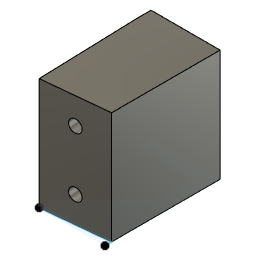
Wanhao-dub-D6-switchholder v3 (Autodesk Fusion 360 design; units mm, degrees)
Autodesk Fusion 360 part; units mm, degrees
note: some values were not read from the file. Set by a fixed rule: which sketch regions a step uses.
sketch "Sketch1" plane through (0, 0, 0) normal (0, 1, 0) x (1, 0, 0)
  line L0 (10, -10) -> (26, -10)
  line L1 (26, -10) -> (26, -50)
  line L2 (26, -50) -> (10, -50)
  line L3 (10, -50) -> (10, -10)
  line L4 (50, -25) -> (70, -25)
  line L5 (70, -25) -> (70, -55)
  line L6 (70, -55) -> (50, -55)
  line L7 (50, -55) -> (50, -25)
  line L8 (70, -25) -> (66, -25)
  line L9 (66, -25) -> (66, -55)
  line L10 (66, -55) -> (70, -55)
  line L11 (70, -55) -> (70, -25)
  dimension "d1" = 16
  dimension "d2" = 40
  dimension "d3" = 20
  dimension "d4" = 30
  dimension "d5" = 4
  dimension "d6" = 16
  constraint horizontal L0
  constraint vertical L1
  constraint horizontal L2
  constraint vertical L3
  constraint horizontal L4
  constraint vertical L5
  constraint horizontal L6
  constraint vertical L7
  constraint horizontal L8
  constraint vertical L9
  constraint horizontal L10
  constraint vertical L11
  measures "d1" distance of L0.start L0.end
  measures "d2" distance of L0.start L2.end
  measures "d3" distance of L4.start L4.end
  measures "d4" distance of L4.start L6.end
  measures "d5" distance of L4.end L8.end
  measures "d6" distance of L7 L9
extrude "Extrude1" add sketch "Sketch1" along normal blind 4 contours L4 L6 L7 L9 makes body 1
extrude "Extrude2" add sketch "Sketch1" along normal blind 35 contours L4 L5 L6 L8 L9 L10 L11 bodies 1
move_body "Move1" bodies 1 to x (1, 0, 0) y (0, 1, 0) z (0, 0, 1) at (-50, 0, -25)
sketch "Sketch2" plane through (16, 0, 0) normal (-1, 0, 0) x (0, 0, 1)
  line L0 (0, 4) -> (30, 4)
  line L1 (30, 4) -> (30, 35)
  line L2 (30, 35) -> (0, 35)
  line L3 (0, 35) -> (0, 4)
  line L4 (0, 35) -> (30, 35)
  line L5 (30, 35) -> (30, 31)
  line L6 (30, 31) -> (0, 31)
  line L7 (0, 31) -> (0, 35)
  dimension "d14" = 4
  constraint horizontal L4
  constraint vertical L5
  constraint horizontal L6
  constraint vertical L7
  constraint coincident L2.end L3.start
  measures "d14" distance of L2.end L6.end
extrude "Extrude3" add sketch "Sketch2" along normal blind 16 contours L1 L2 L3 L4 L5 L6 L7 bodies 1
move_body "Move2" bodies 1 to x (1, 0, 0) y (0, 0, 1) z (0, -1, 0) at (0, 30, 0)
sketch "Sketch3" plane through (0, 30, 0) normal (0, 1, 0) x (-1, 0, 0)
  line L0 (-20, 0) -> (0, 0)
  line L1 (0, 0) -> (0, 4)
  line L2 (0, 4) -> (-16, 4)
  line L3 (-16, 4) -> (-16, 31)
  line L4 (-16, 31) -> (0, 31)
  line L5 (0, 31) -> (0, 35)
  line L6 (0, 35) -> (-20, 35)
  line L7 (-20, 35) -> (-20, 0)
  line L8 (-16, 31) -> (0, 31)
  line L9 (-16, 15) -> (-16, 31)
  line L10 (-16, 15) -> (0, 31)
  dimension "d17" = 16
  constraint horizontal L8
  constraint vertical L9
  constraint coincident L3.end L4.start
  constraint coincident L4.end L5.start
  measures "d17" distance of L3.end L9.start
extrude "Extrude4" add sketch "Sketch3" against normal blind 30 separate body contours L3 L4 L8 L9 L10 makes body 2
move_face "OffsetFaces1" offset 1 1 faces at (0, 10, 1.3333) on bodies 1
sketch "Sketch4" plane through (0, 0, 4) normal (0, 0, 1) x (1, 0, 0)
  line L0 (16, 30) -> (-1, 30)
  line L1 (-1, 30) -> (-1, 0)
  line L2 (-1, 0) -> (16, 0)
  line L3 (16, 0) -> (16, 30)
  line L4 (-1, 30) -> (2, 30)
  line L5 (2, 30) -> (2, 0)
  line L6 (2, 30) -> (2, 26)
  line L7 (2, 26) -> (2, 7)
  circle A0 centre (2, 26) radius 1.5
  circle A1 centre (2, 7) radius 1.5
  dimension "d21" = 3
  dimension "d22" = 4
  dimension "d23" = 19
  dimension "d24" = 3
  dimension "d25" = 3
  constraint coincident L0.end L1.start
  constraint perpendicular L1 L4
  constraint coincident L2 L5.end
  constraint perpendicular L2 L5
  constraint perpendicular L4 L6
  constraint parallel L5 L7
  constraint coincident L6.end L7.start
  constraint coincident L7.end A1.centre
  measures "d21" distance of L0.end L4.end
  measures "d22" distance of L4.end L6.end
  measures "d23" distance of L6.end L7.end
  measures "d24" diameter of A0
  measures "d25" diameter of A1
extrude "Extrude5" cut sketch "Sketch4" against normal blind 6.6 contours L5 L6 L7 A0 | L5 L6 L7 A0 | L5 L7 A1 | L5 L7 A1 bodies 1
sketch "Sketch5" plane through (0, 30, 0) normal (0, 1, 0) x (-1, 0, 0)
  line L0 (-20, 0) -> (1, 0)
  line L1 (1, 0) -> (1, 4)
  line L2 (1, 4) -> (-16, 4)
  line L3 (-16, 4) -> (-16, 31)
  line L4 (-16, 31) -> (0, 31)
  line L5 (0, 31) -> (0, 35)
  line L6 (0, 35) -> (-20, 35)
  line L7 (-20, 35) -> (-20, 0)
  line L8 (-20, 0) -> (0, 0)
  line L9 (0, 35) -> (-20, 35)
  line L10 (-20, 35) -> (-20, 0)
  line L11 (1, 4) -> (0, 35)
  constraint horizontal L8
  constraint horizontal L9
  constraint vertical L10
  constraint coincident L5.end L6.start
  constraint coincident L0.start L7.end
  constraint coincident L1.end L2.start
extrude "Extrude6" add sketch "Sketch5" along normal blind 4 bodies 1 2
sketch "Sketch6" plane through (0, 30, 0) normal (0, -1, 0) x (1, 0, 0)
  line L0 (-1, 4) -> (16, 4)
  line L1 (16, 4) -> (16, 15)
  line L2 (16, 15) -> (0, 31)
  line L3 (0, 31) -> (0, 35)
  line L4 (0, 35) -> (-1, 4)
  line L5 (16, 15) -> (-5.2132, 36.2132)
  dimension "d30" = 30
  constraint coincident L1.end L2.start
  constraint parallel L2 L5
  measures "d30" distance of L1.end L5.end
extrude "Extrude7" add sketch "Sketch6" along normal blind 30 contours L3 L4 L5 bodies 1
sketch "Sketch7" plane through (0, 0, 0) normal (0, -1, 0) x (1, 0, 0)
  line L0 (-1, 0) -> (20, 0)
  line L1 (20, 0) -> (20, 35)
  line L2 (20, 35) -> (0, 35)
  line L3 (0, 35) -> (-0.125, 31.125)
  line L4 (-0.125, 31.125) -> (16, 15)
  line L5 (16, 15) -> (16, 4)
  line L6 (16, 4) -> (-1, 4)
  line L7 (-1, 4) -> (-1, 0)
sketch "Sketch8" plane through (0, 0, 35) normal (0, 0, 1) x (1, 0, 0)
  line L0 (20, 0) -> (20, 34)
  line L1 (20, 34) -> (0, 34)
  line L2 (0, 34) -> (0, 0)
  line L3 (0, 0) -> (20, 0)
  line L4 (10, 34) -> (10, 0)
  line L5 (10, 34) -> (10, 26)
  line L6 (10, 26) -> (14, 26)
  line L7 (10, 0) -> (10, 8)
  circle A0 centre (10, 8) radius 2.1
  circle A1 centre (10, 26) radius 2.1
  dimension "d33" = 8
  dimension "d34" = 4.2
  dimension "d35" = 4.2
  constraint midpoint L1 L4.start
  constraint midpoint L3 L4.end
  constraint coincident L4 L5.end
  constraint perpendicular L1 L5
  constraint perpendicular L4 L6
  constraint perpendicular L3 L7
  constraint coincident L7.end A0.centre
  constraint coincident L5.end L6.start
  measures "d33" distance of L4.end L7.end
  measures "d34" diameter of A0
  measures "d35" diameter of A1
extrude "Extrude8" cut sketch "Sketch8" against normal blind 29 contours L4 L7 A0 | L4 L7 A0 | L4 L5 L6 A1 | L4 L5 A1 | L4 L6 A1 bodies 1
delete_face "DeleteFace1" 1 faces at (9.4653, 10.0308, 26.0443) on bodies 1
delete_face "DeleteFace2" 1 faces at (9.4653, 28.0308, 26.0443) on bodies 1
sketch "Sketch9" plane through (0, 0, 0) normal (0, -1, 0) x (1, 0, 0)
  line L0 (20, 35) -> (20, 33)
  line L1 (20, 33) -> (0, 35)
  point P0 (20, 35)
  point P1 (0, 35)
  dimension "d38" = 2
  constraint coincident P0 L0.start
  constraint coincident P1 L1.end
  measures "d38" distance of P0 L0.end
sketch "Sketch10" plane through (0, 0, 0) normal (0, -1, 0) x (1, 0, 0)
  line L0 (0, 35) -> (20, 33)
  line L1 (20, 33) -> (20, 35)
  line L2 (20, 35) -> (0, 35)
  point P0 (0, 35)
  point P1 (20, 33)
  constraint coincident P0 L0.start
  constraint coincident P1 L0.end
  constraint perpendicular L1 L2
extrude "Extrude9" cut sketch "Sketch10" against normal blind 52 bodies 1
sketch "Sketch11" plane through (3.4653, 0, 34.6535) normal (0.099504, 0, 0.995037) x (0.995037, 0, -0.099504)
  line L0 (16.6171, 34) -> (-3.4826, 34)
  line L1 (-3.4826, 34) -> (-3.4826, 0)
  line L2 (-3.4826, 0) -> (16.6171, 0)
  line L3 (16.6171, 0) -> (16.6171, 34)
  line L4 (6.5672, 34) -> (6.5672, 0)
  line L5 (6.5672, 0) -> (6.5672, 18)
  line L6 (6.5672, 34) -> (6.5672, 26)
  line L7 (6.5672, 0) -> (6.5672, 8)
  circle A0 centre (6.5672, 8) radius 2
  circle A1 centre (6.5672, 26) radius 2
  dimension "d41" = 8
  dimension "d42" = 8
  dimension "d43" = 4
  dimension "d44" = 4
  constraint midpoint L0 L4.start
  constraint midpoint L2 L4.end
  constraint coincident L4 L5.end
  constraint perpendicular L2 L5
  constraint perpendicular L0 L6
  constraint parallel L4 L7
  constraint coincident L7.end A0.centre
  constraint coincident L6.end A1.centre
  measures "d41" distance of L4.start L6.end
  measures "d42" distance of L4.end L7.end
  measures "d43" diameter of A0
  measures "d44" diameter of A1
extrude "Extrude10" cut sketch "Sketch11" against normal blind 26 contours L4 L6 A1 | L4 L6 A1 | L4 L5 L7 A0 | L4 L5 L7 A0 bodies 1
delete_face "DeleteFace3" 1 faces at (11.5359, 8.1578, 29.3215) on bodies 1
delete_face "DeleteFace4" 1 faces at (11.5359, 26.1578, 29.3215) on bodies 1
sketch "Sketch12" plane through (3.4653, 0, 34.6535) normal (0.099504, 0, 0.995037) x (0.995037, 0, -0.099504)
  line L0 (16.6171, 34) -> (-3.4826, 34)
  line L1 (-3.4826, 34) -> (-3.4826, 0)
  line L2 (-3.4826, 0) -> (16.6171, 0)
  line L3 (16.6171, 0) -> (16.6171, 34)
  line L4 (6.5672, 34) -> (6.5672, 0)
  line L5 (6.5672, 0) -> (6.5672, 8)
  line L6 (6.5672, 34) -> (6.5672, 26)
  circle A0 centre (6.5672, 26) radius 1.9
  circle A1 centre (6.5672, 8) radius 1.9
  dimension "d47" = 8
  dimension "d48" = 8
  dimension "d49" = 3.8
  dimension "d50" = 3.8
  constraint midpoint L0 L4.start
  constraint midpoint L2 L4.end
  constraint perpendicular L2 L5
  constraint perpendicular L0 L6
  constraint coincident L6.end A0.centre
  constraint coincident L5.end A1.centre
  measures "d47" distance of L4.end L5.end
  measures "d48" distance of L4.start L6.end
  measures "d49" diameter of A0
  measures "d50" diameter of A1
extrude "Extrude11" cut sketch "Sketch12" against normal blind 16 contours L4 L6 A0 | L4 L6 A0 | L4 L5 A1 | L4 L5 A1 bodies 1
